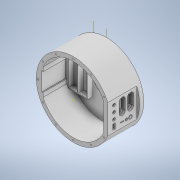
# Autodesk Inventor part: enclosure
Saved by Autodesk Inventor 2020.3 (Build 243373000, 373)
## iProperties
Created: 2020-11-01
Part Number: enclosure
Material: Generic
Document SubType Name: Modeling
Designer: Martijn
Density: 1 g/cm^3
Appearance: Default
Author: Martijn
Autodesk Inventor part; units mm, degrees
ref_plane "YZ Plane" through (0, 0, 0) normal (1, 0, 0) x (0, 1, 0)
ref_plane "XZ Plane" through (0, 0, 0) normal (0, 1, 0) x (-1, 0, 0)
ref_plane "XY Plane" through (0, 0, 0) normal (0, 0, 1) x (1, 0, 0)
sketch "Sketch1" plane through (0, 0, 0) normal (0, 0, 1) x (1, 0, 0)
  circle A0 centre (0, 0) radius 90
  circle A1 centre (0, 0) radius 21
  dimension "d0" = 180
  dimension "d3" = 42
  constraints: 2 centre point, 2 coincident
  measures "d0" diameter of A0
  measures "d3" diameter of A1
extrude "Extrusion1" add sketch "Sketch1" along normal blind 10
sketch "Sketch2" plane through (0, 0, 10) normal (0, 0, 1) x (1, 0, 0)
  arc A0 (82.9156, 35) -> (82.9156, -35) centre (0, 0) ccw
  line L0 (82.9156, 35) -> (82.9156, -35)
  line L1 (0, -140) -> (0, 140) projected
  arc A1 (72.9156, 32.9137) -> (72.9156, -32.9137) centre (0, 0) ccw
  circle A2 centre (0, 0) radius 90 projected
  line L2 (72.9156, 32.9137) -> (72.9156, -32.9137)
  dimension "d4" = 70
  dimension "d5" = 90
  dimension "d7" = 10
  dimension "d34" = 10
  constraints: 4 end point, 4 point on circle, 2 centre point, 2 coincident, 2 parallel, 1 vertical
  measures "d4" distance of L0.start L0.end
  measures "d5" radius of A0
  measures "d7" distance between parallel lines of L0 L2
  measures "d34" radial gap between concentric circles of A1 A0
extrude "Extrusion2" add sketch "Sketch2" along normal blind 70 contours L0 A0 L1 A1 L2 | L1 A1 A0
sketch "Sketch5" plane through (0, 0, 10) normal (0, 0, 1) x (1, 0, 0)
  line L0 (-2.6238, 52) -> (-2.6238, 56)
  line L1 (2.7762, 52) -> (2.7762, 56)
  arc A0 (2.7762, 56) -> (-2.6238, 56) centre (0.0762, 56) ccw
  arc A1 (-2.6238, 52) -> (2.7762, 52) centre (0.0762, 52) ccw
  line L2 (-2.6238, 54) -> (2.7762, 54)
  point P0 (0, 0)
  point P1 (0.0762, 54)
  dimension "d128" = 2.7
  dimension "d129" = 54
  dimension "d130" = 4
  constraints: 7 end point, 4 point on circle, 3 midpoint, 2 centre point, 2 vertical
  measures "d128" radius of A1
  measures "d129" distance of point (0, 0) point (0.076, 54)
  measures "d130" distance of L0.start L0.end
extrude "Extrusion4" cut sketch "Sketch5" against normal blind 10
sketch "Sketch8" plane through (82.9156, -35, 10) normal (1, 0, 0) x (0, 0, -1)
  line L0 (-57.95, 6.2) -> (-52.05, 6.2)
  line L1 (-52.05, 6.2) -> (-52.05, 18.8)
  line L2 (-52.05, 18.8) -> (-57.95, 18.8)
  line L3 (-57.95, 18.8) -> (-57.95, 6.2)
  circle A0 centre (-55, 27.5) radius 3.5
  circle A1 centre (-55, 42.5) radius 3.5
  circle A2 centre (-55, 57.5) radius 3.5
  line L4 (-35, 12.5) -> (-52.05, 12.5)
  line L5 (0, 70) -> (-70, 70) projected
  line L6 (-55, 57.5) -> (-55, 42.5)
  line L7 (-55, 42.5) -> (-55, 27.5)
  line L8 (-55, 27.5) -> (-55, 12.5)
  line L9 (-70, 0) -> (-70, 70) projected
  line L10 (-57.95, 12.5) -> (-52.05, 12.5)
  circle A3 centre (-25, 12.5) radius 3
  line L11 (-25, 12.5) -> (-35, 12.5)
  point P0 (10, 35)
  dimension "d35" = 5.9
  dimension "d36" = 12.6
  dimension "d37" = 7
  dimension "d38" = 7
  dimension "d39" = 7
  dimension "d41" = 15
  dimension "d42" = 15
  dimension "d43" = 15
  dimension "d44" = 12.5
  dimension "d45" = 15
  dimension "d46" = 2.95
  dimension "d47" = 20
  dimension "d64" = 6
  dimension "d66" = 30
  constraints: 20 end point, 4 centre point, 3 collinear, 3 midpoint, 2 horizontal, 2 parallel, 1 perpendicular, 1 point on line, 1 vertical
  measures "d35" distance of L0.start L0.end
  measures "d36" distance of L2.end L0.start
  measures "d37" diameter of A0
  measures "d38" diameter of A1
  measures "d39" diameter of A2
  measures "d41" distance of L6.end L6.start
  measures "d42" distance of L6.end L7.end
  measures "d43" vertical distance of L7.end L4.end
  measures "d44" distance from line of L5 L6.start
  measures "d45" distance from line of L9 L8.end
  measures "d46" distance from line of L3 L8.end
  measures "d47" distance of L8.end L4.start
  measures "d64" diameter of A3
  measures "d66" distance of L11.start L8.end
extrude "Extrusion7" cut sketch "Sketch8" against normal up to surface (10 mm away)
sketch "Sketch9" plane through (82.9156, -35, 10) normal (1, 0, 0) x (0, 0, -1)
  arc A0 (-42.4, 33) -> (-27.6, 33) centre (-35, 33) ccw
  line L0 (-42.4, 33) -> (-42.4, 57)
  arc A1 (-27.6, 57) -> (-42.4, 57) centre (-35, 57) ccw
  line L1 (-27.6, 33) -> (-27.6, 57)
  line L2 (-42.4, 45) -> (-27.6, 45)
  line L3 (0, 70) -> (-70, 70) projected
  circle A2 centre (-55, 27.5) radius 3.5 projected
  point P0 (10, 35)
  dimension "d50" = 14.8
  dimension "d51" = 24
  dimension "d52" = 25
  dimension "d53" = 20
  constraints: 6 end point, 4 point on circle, 4 tangent, 2 centre point, 2 midpoint, 2 vertical
  measures "d50" distance between parallel lines of L1 L0
  measures "d51" distance of A0.centre A1.centre
  measures "d52" distance between parallel lines of L3 L2
  measures "d53" horizontal distance of A2.centre A0.centre
extrude "Extrusion8" cut sketch "Sketch9" against normal blind 5 contours L0 L2 L1 A0 | L0 A1 L1 L2
sketch "Sketch11" plane through (77.9156, -35, 10) normal (1, 0, 0) x (0, 0, -1)
  circle A0 centre (-35, 30.5) radius 1.35
  circle A1 centre (-35, 59.5) radius 1.35
  line L0 (-35, 30.5) -> (-35, 59.5)
  line L1 (-70, -45) -> (-70, 115) projected
  line L2 (-42.4, 33) -> (-42.4, 57) projected
  line L3 (-42.4, 45) -> (-35, 45)
  line L4 (-35, 45) -> (-27.6, 45)
  line L5 (-27.6, 57) -> (-27.6, 33) projected
  line L6 (-42.4, 33) -> (-27.6, 33)
  line L7 (-27.6, 33) -> (-27.6, 57)
  line L8 (-27.6, 57) -> (-42.4, 57)
  line L9 (-42.4, 57) -> (-42.4, 33)
  point P0 (10, 35)
  point P1 (-70, 2.0863)
  point P2 (-70, 67.9137)
  point P3 (-35, 57)
  dimension "d56" = 29
  dimension "d57" = 2.7
  dimension "d58" = 2.7
  constraints: 14 end point, 4 parallel, 3 midpoint, 2 centre point, 2 perpendicular, 1 collinear, 1 horizontal
  measures "d56" distance of L0.start L0.end
  measures "d57" diameter of A0
  measures "d58" diameter of A1
extrude "Extrusion9" cut sketch "Sketch11" against normal up to surface (5 mm away)
pattern_linear "Rectangular Pattern1" count 2 spacing 20 along (0, 0, -1) of "Extrusion8", "Extrusion9"
sketch "Sketch12" plane through (82.9156, -35, 10) normal (1, 0, 0) x (0, 0, -1)
  point P0 (10, 35)
sketch "Sketch13" plane through (72.9156, -32.9137, 10) normal (-1, 0, 0) x (0, 0, 1)
  line L0 (18.5, 4.4137) -> (31.5, 4.4137)
  line L1 (31.5, 4.4137) -> (31.5, 16.4137)
  line L2 (31.5, 16.4137) -> (18.5, 16.4137)
  line L3 (18.5, 16.4137) -> (18.5, 4.4137)
  circle A0 centre (25, 10.4137) radius 3 projected
  point P0 (-10, 32.9137)
  dimension "d67" = 6.5
  dimension "d68" = 6.5
  dimension "d69" = 6
  dimension "d70" = 6
  constraints: 8 end point, 2 parallel, 1 horizontal, 1 perpendicular
  measures "d67" distance from line of L3 A0.centre
  measures "d68" distance from line of L1 A0.centre
  measures "d69" distance from line of A0.centre L2
  measures "d70" distance from line of A0.centre L0
extrude "Extrusion10" cut sketch "Sketch13" against normal blind 5
sketch "Sketch14" plane through (72.9156, -32.9137, 10) normal (-1, 0, 0) x (0, 0, 1)
  circle A0 centre (55, 25.4137) radius 5
  circle A1 centre (55, 40.4137) radius 5
  circle A2 centre (55, 55.4137) radius 5
  circle A3 centre (55, 25.4137) radius 3.5 projected
  circle A4 centre (55, 40.4137) radius 3.5 projected
  circle A5 centre (55, 55.4137) radius 3.5 projected
  point P0 (-10, 32.9137)
  dimension "d73" = 10
  dimension "d74" = 10
  dimension "d75" = 10
  constraints: 3 centre point, 3 concentric
  measures "d73" diameter of A0
  measures "d74" diameter of A1
  measures "d75" diameter of A2
extrude "Extrusion11" cut sketch "Sketch14" against normal blind 7
sketch "Sketch15" plane through (82.9156, -35, 10) normal (1, 0, 0) x (0, 0, -1)
  line L0 (-39, 11.75) -> (-31, 11.75)
  line L1 (-31, 11.75) -> (-31, 13.25)
  line L2 (-31, 13.25) -> (-39, 13.25)
  line L3 (-39, 13.25) -> (-39, 11.75)
  circle A0 centre (-15, 12.5) radius 3.5
  circle A1 centre (-15, 12.5) radius 4.5
  circle A2 centre (-25, 12.5) radius 3 projected
  line L4 (-25, 12.5) -> (-15, 12.5)
  line L5 (-25, 12.5) -> (-35, 12.5)
  line L6 (-35, 13.25) -> (-35, 11.75)
  point P0 (10, 35)
  dimension "d78" = 1.5
  dimension "d79" = 8
  dimension "d80" = 7
  dimension "d81" = 9
  dimension "d82" = 10
  dimension "d83" = 10
  constraints: 14 end point, 3 midpoint, 2 centre point, 2 horizontal, 2 parallel, 1 coincident, 1 collinear, 1 perpendicular
  measures "d78" distance between parallel lines of L0 L2
  measures "d79" distance of L0.start L0.end
  measures "d80" diameter of A0
  measures "d81" diameter of A1
  measures "d82" distance of L4.start L5.end
  measures "d83" distance of L4.start A0.centre
extrude "Extrusion12" cut sketch "Sketch15" against normal blind 1 contours L3 L2 L6 L0 | L6 L5 L1 L0 | L6 L2 L1 L5 | A1
sketch "Sketch16" plane through (0, 0, 10) normal (0, 0, 1) x (1, 0, 0)
  line L0 (-46.2, -38.1943) -> (-25, -38.1943)
  line L1 (-25, -38.1943) -> (-25, 37.4057)
  line L2 (-25, 37.4057) -> (-46.2, 37.4057)
  line L3 (-46.2, 37.4057) -> (-46.2, -38.1943)
  line L4 (-69.4, -38.1943) -> (-48.2, -38.1943)
  line L5 (-48.2, -38.1943) -> (-48.2, 37.4057)
  line L6 (-48.2, 37.4057) -> (-69.4, 37.4057)
  line L7 (-69.4, 37.4057) -> (-69.4, -38.1943)
  line L8 (-71.4, -40.1943) -> (-23, -40.1943)
  line L9 (-23, -40.1943) -> (-23, 39.4057)
  line L10 (-23, 39.4057) -> (-71.4, 39.4057)
  line L11 (-71.4, 39.4057) -> (-71.4, -40.1943)
  point P0 (0, 0)
  dimension "d86" = 21.2
  dimension "d87" = 21.2
  dimension "d88" = 75.6
  dimension "d89" = 75.6
  dimension "d90" = 2
  dimension "d91" = 2
  dimension "d92" = 2
  dimension "d93" = 2
  dimension "d94" = 2
  dimension "d95" = 23
  constraints: 24 end point, 6 parallel, 3 horizontal, 3 perpendicular, 1 point on line
  measures "d86" distance between parallel lines of L1 L3
  measures "d87" distance between parallel lines of L5 L7
  measures "d88" distance between parallel lines of L0 L2
  measures "d89" distance between parallel lines of L4 L6
  measures "d90" distance between parallel lines of L3 L5
  measures "d91" distance between parallel lines of L9 L1
  measures "d92" distance between parallel lines of L0 L8
  measures "d93" distance between parallel lines of L7 L11
  measures "d94" distance between parallel lines of L6 L10
  measures "d95" distance from line of L9 point (0, 0)
extrude "Extrusion13" add sketch "Sketch16" along normal blind 13
sketch "Sketch17" plane through (-46.2, -38.1943, 10) normal (0, 1, 0) x (1, 0, 0)
  circle A0 centre (19.7, -1.5) radius 1
  line L0 (21.2, 0) -> (21.2, -13) projected
  line L1 (0, 0) -> (21.2, 0) projected
  circle A1 centre (-21.7, -1.5) radius 1
  line L2 (-23.2, 0) -> (-23.2, -13) projected
  line L3 (-23.2, 0) -> (-2, 0) projected
  point P0 (46.2, 10)
  dimension "d98" = 2
  dimension "d99" = 1.5
  dimension "d100" = 1.5
  dimension "d101" = 2
  dimension "d102" = 1.5
  dimension "d103" = 1.5
  constraints: 2 centre point
  measures "d98" diameter of A0
  measures "d99" distance from line of L0 A0.centre
  measures "d100" distance from line of L1 A0.centre
  measures "d101" diameter of A1
  measures "d102" distance from line of A1.centre L2
  measures "d103" distance from line of L3 A1.centre
extrude "Extrusion14" cut sketch "Sketch17" against normal blind 2
sketch "Sketch18" plane through (-46.2, 37.4057, 10) normal (0, -1, 0) x (1, 0, 0)
  circle A0 centre (1.5, 1.5) radius 1
  circle A1 centre (-3.5, 1.5) radius 1
  line L0 (21.2, 0) -> (0, 0) projected
  line L1 (0, 0) -> (0, 13) projected
  line L2 (-2, 0) -> (-2, 13) projected
  line L3 (-2, 0) -> (-23.2, 0) projected
  point P0 (46.2, -10)
  dimension "d106" = 2
  dimension "d107" = 2
  dimension "d108" = 1.5
  dimension "d109" = 1.5
  dimension "d110" = 1.5
  dimension "d111" = 1.5
  constraints: 2 centre point
  measures "d106" diameter of A1
  measures "d107" diameter of A0
  measures "d108" distance from line of L0 A0.centre
  measures "d109" distance from line of A0.centre L1
  measures "d110" distance from line of L2 A1.centre
  measures "d111" distance from line of L3 A1.centre
extrude "Extrusion15" cut sketch "Sketch18" against normal blind 2
sketch "Sketch19" plane through (0, 0, 80) normal (0, 0, 1) x (1, 0, 0)
  circle A0 centre (73.6122, -42.5) radius 1.6
  line L0 (73.6122, -42.5) -> (0, 0)
  line L1 (-126, 0) -> (126, 0) projected
  dimension "d114" = 85
  dimension "d115" = 3.2
  dimension "d116" = 30
  constraints: 2 end point, 1 centre point
  measures "d114" distance of L0.start L0.end
  measures "d115" diameter of A0
  measures "d116" angle of L1 L0
extrude "Extrusion16" cut sketch "Sketch19" against normal blind 100
sketch "Sketch20" plane through (0, 0, 0) normal (0, 0, -1) x (-1, 0, 0)
  circle A0 centre (-73.6122, -42.5) radius 3
  circle A1 centre (-73.6122, -42.5) radius 1.6 projected
  point P0 (0, 0)
  dimension "d122" = 6
  constraints: 1 centre point, 1 concentric
  measures "d122" diameter of A0
extrude "Extrusion17" cut sketch "Sketch20" against normal blind 54
pattern_circular "Circular Pattern2" count 11 over 300 about axis through (0, 0, 0) along (0, 0, -1) of "Extrusion17", "Extrusion16"
sketch "Sketch22" plane through (0, 0, 10) normal (0, 0, 1) x (1, 0, 0)
  line L0 (25, -38.1943) -> (46.2, -38.1943)
  line L1 (46.2, -38.1943) -> (46.2, 37.4057)
  line L2 (46.2, 37.4057) -> (25, 37.4057)
  line L3 (25, 37.4057) -> (25, -38.1943)
  line L4 (23, -40.1943) -> (48.2, -40.1943)
  line L5 (48.2, -40.1943) -> (48.2, 39.4057)
  line L6 (48.2, 39.4057) -> (23, 39.4057)
  line L7 (23, 39.4057) -> (23, -40.1943)
  line L8 (-69.1695, -40.1943) -> (-23, -40.1943) projected
  point P0 (0, 0)
  dimension "d131" = 21.2
  dimension "d132" = 75.6
  dimension "d134" = 2
  dimension "d135" = 2
  dimension "d136" = 2
  dimension "d137" = 2
  dimension "d138" = 23
  constraints: 16 end point, 4 parallel, 2 horizontal, 2 perpendicular, 1 collinear
  measures "d131" distance between parallel lines of L1 L3
  measures "d132" distance between parallel lines of L2 L0
  measures "d134" distance between parallel lines of L3 L7
  measures "d135" distance between parallel lines of L0 L4
  measures "d136" distance between parallel lines of L5 L1
  measures "d137" distance between parallel lines of L6 L2
  measures "d138" distance from line of L7 point (0, 0)
extrude "Extrusion18" add sketch "Sketch22" along normal up to surface (13 mm away)
sketch "Sketch23" plane through (0, 0, 10) normal (0, 0, 1) x (1, 0, 0)
  arc A0 (-17.0238, 36.5) -> (-13.8238, 36.5) centre (-15.4238, 36.5) ccw
  line L0 (-17.0238, 36.5) -> (-17.0238, 40.5)
  arc A1 (-13.8238, 40.5) -> (-17.0238, 40.5) centre (-15.4238, 40.5) ccw
  line L1 (-13.8238, 40.5) -> (-13.8238, 36.5)
  line L2 (-17.0238, 38.5) -> (-13.8238, 38.5)
  line L3 (-2.6238, 56) -> (-2.6238, 52) projected
  line L4 (-2.6238, 54) -> (2.7762, 54)
  line L5 (2.7762, 56) -> (2.7762, 52) projected
  point P0 (0, 0)
  point P1 (-15.4238, 38.5)
  point P2 (0.0762, 54)
  dimension "d141" = 1.6
  dimension "d142" = 4
  dimension "d143" = 15.5
  dimension "d144" = 15.5
  constraints: 8 end point, 6 midpoint, 4 point on circle, 4 tangent, 2 centre point, 2 vertical, 1 horizontal
  measures "d141" radius of A1
  measures "d142" distance of L0.start L0.end
  measures "d143" horizontal distance of point (0.076, 54) point (-15.424, 38.5)
  measures "d144" horizontal distance of point (0.076, 54) point (-15.424, 38.5)
extrude "Extrusion19" cut sketch "Sketch23" against normal blind 10
pattern_linear "Rectangular Pattern2" count 2 spacing 31 along (1, 0, 0) count 2 spacing 31 along (0, 1, 0) of "Extrusion19"
sketch "Sketch24" plane through (25, -38.1943, 10) normal (0, 1, 0) x (1, 0, 0)
  circle A0 centre (1.5, -1.5) radius 1
  line L0 (0, 0) -> (0, -13) projected
  line L1 (0, 0) -> (21.2, 0) projected
  point P0 (-25, 10)
  dimension "d153" = 2
  dimension "d154" = 1.5
  dimension "d155" = 1.5
  constraints: 1 centre point
  measures "d153" diameter of A0
  measures "d154" distance from line of L0 A0.centre
  measures "d155" distance from line of L1 A0.centre
extrude "Extrusion20" cut sketch "Sketch24" against normal blind 10
sketch "Sketch25" plane through (25, 37.4057, 10) normal (0, -1, 0) x (1, 0, 0)
  circle A0 centre (19.7, 1.5) radius 1
  line L0 (21.2, 0) -> (21.2, 13) projected
  line L1 (21.2, 0) -> (0, 0) projected
  point P0 (-25, -10)
  dimension "d158" = 2
  dimension "d159" = 1.5
  dimension "d160" = 1.5
  constraints: 1 centre point
  measures "d158" diameter of A0
  measures "d159" distance from line of L0 A0.centre
  measures "d160" distance from line of L1 A0.centre
extrude "Extrusion21" cut sketch "Sketch25" against normal blind 10
sketch "Sketch28" plane through (0, 0, 80) normal (0, 0, 1) x (1, 0, 0)
  point P0 (0, 0)
sketch "Sketch29" plane through (0, 0, 80) normal (0, 0, 1) x (1, 0, 0)
  arc A0 (72.9156, 32.9137) -> (72.9156, -32.9137) centre (0, 0) ccw projected
  line L0 (-76.7266, -22.65) -> (-76.7266, 22.65)
  line L1 (-76.7266, -22.65) -> (-75.3266, -22.65)
  line L2 (-75.3266, -22.65) -> (-75.3266, -21.65)
  line L3 (-75.3266, -21.65) -> (-73.3266, -21.65)
  line L4 (-73.3266, -21.65) -> (-73.3266, -31.9876)
  line L5 (-76.7266, 22.65) -> (-75.3266, 22.65)
  line L6 (-75.3266, 22.65) -> (-75.3266, 21.65)
  line L7 (-75.3266, 21.65) -> (-73.3266, 21.65)
  line L8 (-73.3266, 21.65) -> (-73.3266, 31.9876)
  arc A1 (-73.3266, 31.9876) -> (-76.7266, 22.65) centre (0, 0) ccw
  arc A2 (-76.7266, 22.65) -> (-76.7266, -22.65) centre (0, 0) ccw
  arc A3 (-76.7266, -22.65) -> (-73.3266, -31.9876) centre (0, 0) ccw
  dimension "d176" = 45.3
  dimension "d177" = 1.4
  dimension "d178" = 2
  dimension "d179" = 1
  dimension "d180" = 1
  dimension "d181" = 1.4
  dimension "d182" = 2
  constraints: 18 end point, 10 point on circle, 5 perpendicular, 3 centre point, 3 coincident, 2 horizontal, 2 vertical
  measures "d176" distance of L0.start L0.end
  measures "d177" distance between parallel lines of L0 L2
  measures "d178" distance between parallel lines of L4 L2
  measures "d179" distance between parallel lines of L1 L3
  measures "d180" distance from line of L6.end L5
  measures "d181" distance between parallel lines of L0 L6
  measures "d182" distance of L6.end L7.end
extrude "Extrusion23" add sketch "Sketch29" against normal up to surface (70 mm away)
sketch "Sketch30" plane through (0, 0, 10) normal (0, 0, 1) x (1, 0, 0)
  line L0 (-71.4, -36.0838) -> (-71.4, 36.0838) projected
  arc A0 (-71.4, 36.0838) -> (-71.4, -36.0838) centre (0, 0) ccw
  line L1 (-71.4, -36.0838) -> (-71.4, 36.0838)
  constraints: 2 end point, 2 point on circle, 1 centre point, 1 coincident, 1 vertical
extrude "Extrusion24" add sketch "Sketch30" along normal up to surface (13 mm away)
sketch "Sketch31" plane through (0, 0, 0) normal (0, 0, -1) x (-1, 0, 0)
  line L0 (-19.0762, 36.5) -> (-19.0762, 40.5)
  arc A0 (-12.0762, 40.5) -> (-19.0762, 40.5) centre (-15.5762, 40.5) ccw
  line L1 (-12.0762, 40.5) -> (-12.0762, 36.5)
  arc A1 (-19.0762, 36.5) -> (-12.0762, 36.5) centre (-15.5762, 36.5) ccw
  line L2 (-17.1762, 36.5) -> (-17.1762, 40.5) projected
  arc A2 (-13.9762, 40.5) -> (-17.1762, 40.5) centre (-15.5762, 40.5) ccw projected
  arc A3 (-17.1762, 36.5) -> (-13.9762, 36.5) centre (-15.5762, 36.5) ccw projected
  point P0 (0, 0)
  dimension "d187" = 3.5
  constraints: 4 end point, 4 point on circle, 4 tangent, 2 centre point, 2 concentric, 2 vertical, 1 parallel
  measures "d187" radius of A1
extrude "Extrusion25" cut sketch "Sketch31" against normal blind 4
pattern_linear "Rectangular Pattern3" count 2 spacing 31 along (0, 1, 0) count 2 spacing 31 along (-1, 0, 0) of "Extrusion25"
sketch "Sketch32" plane through (0, 0, 80) normal (0, 0, 1) x (1, 0, 0)
  point P0 (0, 0)
body "Solid1"
